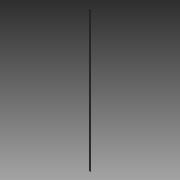
# Autodesk Inventor part: GT2_XY_belting
Saved by Autodesk Inventor 2014 (Build 180170000, 170)
## iProperties
Created: 2013-05-31
Part Number: GT2_XY_belting
Material: Rubber
Document SubType Name: Modeling
Designer: Edward
Density: 0.93 g/cm^3
Description: 550mm GT2 Belting, Cut to length
Vendor: custom
Appearance: Rubber - Black - Version 1.1
Author: Edward
Autodesk Inventor part; units mm, degrees
ref_plane "YZ Plane" through (0, 0, 0) normal (1, 0, 0) x (0, 1, 0)
ref_plane "XZ Plane" through (0, 0, 0) normal (0, 1, 0) x (-1, 0, 0)
ref_plane "XY Plane" through (0, 0, 0) normal (0, 0, 1) x (1, 0, 0)
sketch "Sketch1" plane through (0, 0, 0) normal (0, 0, 1) x (1, 0, 0)
  line L0 (-3, 1) -> (3, 1)
  line L1 (3, 1) -> (3, -1)
  line L2 (3, -1) -> (-3, -1)
  line L3 (-3, -1) -> (-3, 1)
  point P0 (0, 0)
  dimension "d0" = 6
  dimension "d1" = 2
  dimension "d2" = 1
  dimension "d3" = 3
  constraints: 8 end point, 2 parallel, 1 horizontal, 1 perpendicular
  measures "d0" distance of L1.end L2.end
  measures "d1" distance of L0.end L1.end
  measures "d2" distance from line of L0 point (0, 0)
  measures "d3" distance from line of L3 point (0, 0)
extrude "Extrusion1" add sketch "Sketch1" along normal blind 550
equation "\"d2\" = 0.5 * d1"
equation "\"d3\" = 0.5 * d0"
body "Solid1"
